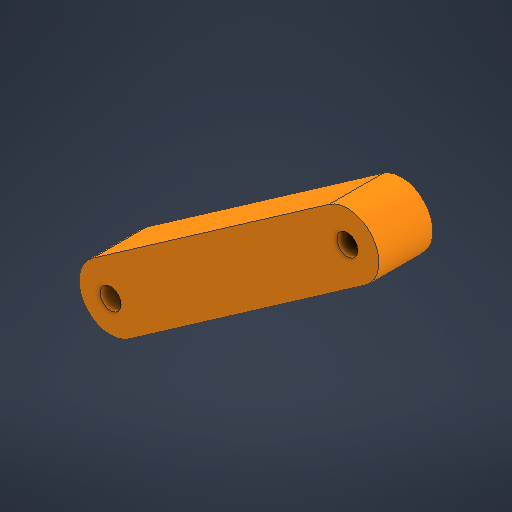
# Autodesk Inventor part: Intermediate
Saved by Autodesk Inventor 2026 (Build 300175000, 175)
## iProperties
Created: 2026-01-04
Part Number: Intermediate
Material: Generic
Document SubType Name: Modeling
Designer: saraswat22
Density: 1 g/cm^3
Appearance: Default
Author: saraswat22
Autodesk Inventor part; units mm, degrees
ref_plane "YZ Plane" through (0, 0, 0) normal (1, 0, 0) x (0, 1, 0)
ref_plane "XZ Plane" through (0, 0, 0) normal (0, 1, 0) x (-1, 0, 0)
ref_plane "XY Plane" through (0, 0, 0) normal (0, 0, 1) x (1, 0, 0)
sketch "Sketch1" plane through (0, 0, 0) normal (0, 0, 1) x (1, 0, 0)
  arc A0 (43.5858, -62.5037) -> (-43.5858, 62.5037) centre (0, 0) ccw
  circle A1 centre (0, 0) radius 25.4
  arc A2 (-614.5778, -335.6666) -> (-527.4062, -460.6741) centre (-570.992, -398.1704) ccw
  circle A3 centre (-570.992, -398.1704) radius 25.4
  line L0 (-614.5778, -335.6666) -> (-43.5858, 62.5037)
  line L1 (-527.4062, -460.6741) -> (43.5858, -62.5037)
  constraints: 4 centre point, 4 end point, 4 point on circle, 4 tangent, 3 coincident, 1 parallel
extrude "Extrusion1" add sketch "Sketch1" along normal blind 130.302
body "Solid1"
